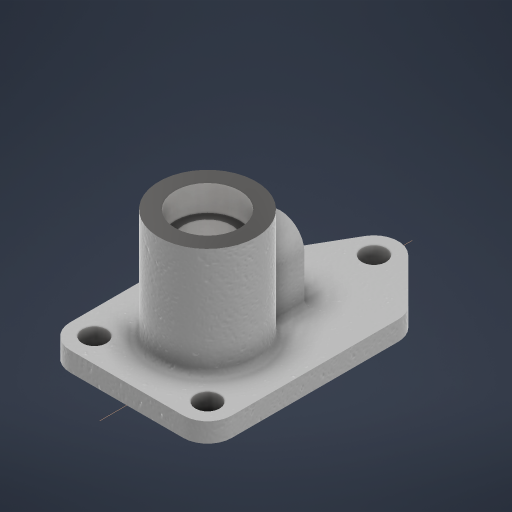
# Autodesk Inventor part: Part1
Saved by Autodesk Inventor 2023 (Build 270158000, 158)
## iProperties
Created: 2022-11-28
Part Number: Part1
Material: Steel, Carbon
Document SubType Name: Modeling
Designer: iusti
Density: 7.85 g/cm^3
Appearance: Textured - Gray
Author: iusti
Autodesk Inventor part; units mm, degrees
note: some values were not read from the file. Chosen so that the rebuilt part matches the saved one: direction of "Hole4".
ref_plane "YZ Plane" through (0, 0, 0) normal (1, 0, 0) x (0, 1, 0)
ref_plane "XZ Plane" through (0, 0, 0) normal (0, 1, 0) x (-1, 0, 0)
ref_plane "XY Plane" through (0, 0, 0) normal (0, 0, 1) x (1, 0, 0)
sketch "Sketch1" plane through (0, 0, 0) normal (0, 1, 0) x (-1, 0, 0)
  line L0 (35, 50) -> (-35, 50)
  line L1 (-50, 35) -> (-50, -68)
  line L2 (-45.6066, -78.6066) -> (-18.6066, -105.6066)
  line L3 (4.9904, -102.5) -> (47.9904, -28.0218)
  line L4 (50, -20.5218) -> (50, 35)
  line L5 (0, -144.3313) -> (0, 86.0129) construction
  arc A0 (-18.6066, -105.6066) -> (4.9904, -102.5) centre (-8, -95) ccw
  arc A1 (47.9904, -28.0218) -> (50, -20.5218) centre (35, -20.5218) ccw
  arc A2 (50, 35) -> (35, 50) centre (35, 35) ccw
  arc A3 (-35, 50) -> (-50, 35) centre (-35, 35) ccw
  arc A4 (-50, -68) -> (-45.6066, -78.6066) centre (-35, -68) ccw
  point P0 (0, 0)
  point P1 (50, 50)
  point P2 (-50, 50)
  point P3 (0, 50)
  dimension "d0" = 100
  dimension "d1" = 50
  dimension "d2" = 135
  dimension "d3" = 15
  dimension "d4" = 42
  dimension "d5" = 145
  dimension "d6" = 30
  dimension "d7" = 15
  constraints: 10 end point, 10 point on circle, 10 tangent, 5 centre point, 5 point on line, 3 equal radius, 2 perpendicular, 1 horizontal, 1 midpoint
  measures "d0" distance of point (50, 50) point (-50, 50)
  measures "d1" distance from line of point (0, 0) L0
  measures "d2" angle of L2 L1
  measures "d3" radius of A0
  measures "d4" distance from line of A0.centre L1
  measures "d5" distance from line of A0.centre L0
  measures "d6" angle of L3 L4
  measures "d7" radius of A1
extrude "Extrusion1" add sketch "Sketch1" along normal blind 12
sketch "Sketch2" plane through (0, 12, 0) normal (0, 1, 0) x (1, 0, 0)
  arc A0 (35, -50) -> (50, -35) centre (35, -35) ccw projected
  arc A1 (-50, -35) -> (-35, -50) centre (-35, -35) ccw projected
  arc A2 (18.6066, 105.6066) -> (-4.9904, 102.5) centre (8, 95) ccw projected
  point P0 (0, 0)
  constraints: 3 coincident
hole "Hole1" at (35, 12, 35) at (-35, 12, 35) at (8, 12, -95) direction (0, -1, 0) diameter 15 end through all
sketch "Sketch3" plane through (0, 12, 0) normal (0, 1, 0) x (1, 0, 0)
  circle A0 centre (0, 0) radius 30
  dimension "d17" = 60
  constraints: 1 centre point, 1 coincident
  measures "d17" diameter of A0
extrude "Extrusion2" add sketch "Sketch3" along normal blind 68
sketch "Sketch5" plane through (0, 0, 0) normal (0, 0, 1) x (1, 0, 0)
  arc A0 (15, 42) -> (-15, 42) centre (0, 42) ccw
  line L0 (15, 42) -> (15, 0)
  line L1 (-15, 42) -> (-15, 0)
  line L2 (15, 0) -> (-15, 0)
  line L3 (-70, 0) -> (70, 0) construction
  point P0 (0, 0)
  dimension "d39" = 30
  dimension "d41" = 42
  constraints: 6 end point, 2 point on circle, 2 tangent, 2 vertical, 1 centre point, 1 collinear, 1 vertical alignment
  measures "d39" diameter of A0
  measures "d41" distance from line of L2 A0.centre
extrude "Extrusion4" add sketch "Sketch5" against normal blind 45
sketch "Sketch6" plane through (0, 80, 0) normal (0, 1, 0) x (1, 0, 0)
  circle A0 centre (0, 0) radius 30 projected
  constraints: 1 coincident
hole "Hole3" at (0, 80, 0) direction (0, -1, 0) diameter 30 end through all counterbore diameter 40 counterbore depth 16
sketch "Sketch7" plane through (0, 0, -45) normal (0, 0, -1) x (-1, 0, 0)
  arc A0 (15, 42) -> (-15, 42) centre (0, 42) ccw projected
  point P0 (0, 0)
  constraints: 1 coincident
hole "Hole4" at (0, 42, -45) direction (0, 0, 1) diameter 16 end up to surface
fillet "Fillet1" radius 4 7 edges at (25.9808, 12, -15) (-15, 12, 25.9808) (15, 12, -35.4904) (-15, 27, -25.9808) (15, 27, -25.9808) (-0.0148, 57, -30) (0, 12, -45)
body "Solid1"
